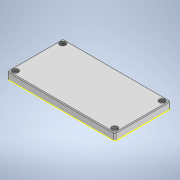
# Autodesk Inventor part: CustomLid_Rev3a
Saved by Autodesk Inventor 2021 (Build 250183000, 183)
## iProperties
Created: 2021-04-06
Part Number: CustomLid_Rev3a
Material: Generic
Document SubType Name: Modeling
Designer: James
Density: 1 g/cm^3
Appearance: Default
Author: James
Autodesk Inventor part; units mm, degrees
ref_plane "YZ Plane" through (0, 0, 0) normal (1, 0, 0) x (0, 1, 0)
ref_plane "XZ Plane" through (0, 0, 0) normal (0, 1, 0) x (-1, 0, 0)
ref_plane "XY Plane" through (0, 0, 0) normal (0, 0, 1) x (1, 0, 0)
sketch "Sketch1" plane through (0, 0, 0) normal (0, 1, 0) x (-1, 0, 0)
  line L0 (103.9624, -60.4464) -> (103.9624, 16.5536) projected
  arc A0 (103.9624, 16.5536) -> (101.9624, 18.5536) centre (101.9624, 16.5536) ccw projected
  line L1 (101.9624, 18.5536) -> (-50.0376, 18.5536) projected
  arc A1 (-50.0376, 18.5536) -> (-52.0376, 16.5536) centre (-50.0376, 16.5536) ccw projected
  line L2 (-52.0376, 16.5536) -> (-52.0376, -60.4464) projected
  arc A2 (-52.0376, -60.4464) -> (-50.0376, -62.4464) centre (-50.0376, -60.4464) ccw projected
  line L3 (-50.0376, -62.4464) -> (101.9624, -62.4464) projected
  arc A3 (101.9624, -62.4464) -> (103.9624, -60.4464) centre (101.9624, -60.4464) ccw projected
  arc A4 (97.8999, -50.5293) -> (92.0453, -56.3839) centre (97.7805, -56.2644) ccw projected
  arc A5 (97.8833, -51.3291) -> (92.8451, -56.3672) centre (97.7805, -56.2644) ccw projected
  circle A6 centre (97.7805, -56.2644) radius 2.5 projected
  arc A7 (97.8999, -50.5293) -> (100.9624, -47.5299) centre (97.9624, -47.5299) ccw projected
  arc A8 (97.8833, -51.3291) -> (101.7624, -47.5299) centre (97.9624, -47.5299) ccw projected
  line L4 (100.9624, 3.6371) -> (100.9624, -47.5299) projected
  line L5 (101.7624, -47.5299) -> (101.7624, 3.6371) projected
  arc A9 (89.046, -60.2464) -> (92.8451, -56.3672) centre (89.046, -56.4464) ccw projected
  arc A10 (89.046, -59.4464) -> (92.0453, -56.3839) centre (89.046, -56.4464) ccw projected
  line L6 (89.046, -59.4464) -> (-37.1211, -59.4464) projected
  line L7 (-37.1211, -60.2464) -> (89.046, -60.2464) projected
  circle A11 centre (-45.8556, -56.2644) radius 2.5 projected
  arc A12 (-40.9203, -56.3672) -> (-45.9584, -51.3291) centre (-45.8556, -56.2644) ccw projected
  arc A13 (-40.1204, -56.3839) -> (-45.9751, -50.5293) centre (-45.8556, -56.2644) ccw projected
  arc A14 (-40.1204, -56.3839) -> (-37.1211, -59.4464) centre (-37.1211, -56.4464) ccw projected
  arc A15 (-40.9203, -56.3672) -> (-37.1211, -60.2464) centre (-37.1211, -56.4464) ccw projected
  arc A16 (-49.0376, -47.5299) -> (-45.9751, -50.5293) centre (-46.0376, -47.5299) ccw projected
  arc A17 (-49.8376, -47.5299) -> (-45.9584, -51.3291) centre (-46.0376, -47.5299) ccw projected
  line L8 (-49.0376, -47.5299) -> (-49.0376, 3.6371) projected
  line L9 (-49.8376, 3.6371) -> (-49.8376, -47.5299) projected
  circle A18 centre (-45.8556, 12.3716) radius 2.5 projected
  arc A19 (-45.9584, 7.4363) -> (-40.9203, 12.4745) centre (-45.8556, 12.3716) ccw projected
  arc A20 (-45.9751, 6.6365) -> (-40.1204, 12.4911) centre (-45.8556, 12.3716) ccw projected
  arc A21 (-45.9584, 7.4363) -> (-49.8376, 3.6371) centre (-46.0376, 3.6371) ccw projected
  arc A22 (-45.9751, 6.6365) -> (-49.0376, 3.6371) centre (-46.0376, 3.6371) ccw projected
  line L10 (-49.0376, -47.5299) -> (-49.0376, 3.6371) projected
  line L11 (-49.8376, 3.6371) -> (-49.8376, -47.5299) projected
  arc A23 (-37.1211, 16.3536) -> (-40.9203, 12.4745) centre (-37.1211, 12.5536) ccw projected
  arc A24 (-37.1211, 15.5536) -> (-40.1204, 12.4911) centre (-37.1211, 12.5536) ccw projected
  line L12 (89.046, 16.3536) -> (-37.1211, 16.3536) projected
  line L13 (-37.1211, 15.5536) -> (89.046, 15.5536) projected
  circle A25 centre (97.7805, 12.3716) radius 2.5 projected
  arc A26 (100.9624, 3.6371) -> (97.8999, 6.6365) centre (97.9624, 3.6371) ccw projected
  arc A27 (101.7624, 3.6371) -> (97.8833, 7.4363) centre (97.9624, 3.6371) ccw projected
  arc A28 (92.8451, 12.4745) -> (97.8833, 7.4363) centre (97.7805, 12.3716) ccw projected
  arc A29 (92.0453, 12.4911) -> (97.8999, 6.6365) centre (97.7805, 12.3716) ccw projected
  arc A30 (92.0453, 12.4911) -> (89.046, 15.5536) centre (89.046, 12.5536) ccw projected
  arc A31 (92.8451, 12.4745) -> (89.046, 16.3536) centre (89.046, 12.5536) ccw projected
  arc A32 (-48.3376, -47.5299) -> (-45.9897, -49.8294) centre (-46.0376, -47.5299) ccw
  arc A33 (-39.4206, -56.3985) -> (-45.9897, -49.8294) centre (-45.8556, -56.2644) ccw
  arc A34 (-39.4206, -56.3985) -> (-37.1211, -58.7464) centre (-37.1211, -56.4464) ccw
  line L14 (-37.1211, -58.7464) -> (89.046, -58.7464)
  arc A35 (89.046, -58.7464) -> (91.3455, -56.3985) centre (89.046, -56.4464) ccw
  arc A36 (97.9145, -49.8294) -> (91.3455, -56.3985) centre (97.7805, -56.2644) ccw
  arc A37 (97.9145, -49.8294) -> (100.2624, -47.5299) centre (97.9624, -47.5299) ccw
  line L15 (100.2624, -47.5299) -> (100.2624, 3.6371)
  arc A38 (100.2624, 3.6371) -> (97.9145, 5.9366) centre (97.9624, 3.6371) ccw
  arc A39 (91.3455, 12.5057) -> (97.9145, 5.9366) centre (97.7805, 12.3716) ccw
  arc A40 (91.3455, 12.5057) -> (89.046, 14.8536) centre (89.046, 12.5536) ccw
  line L16 (89.046, 14.8536) -> (-37.1211, 14.8536)
  arc A41 (-37.1211, 14.8536) -> (-39.4206, 12.5057) centre (-37.1211, 12.5536) ccw
  arc A42 (-45.9897, 5.9366) -> (-39.4206, 12.5057) centre (-45.8556, 12.3716) ccw
  arc A43 (-45.9897, 5.9366) -> (-48.3376, 3.6371) centre (-46.0376, 3.6371) ccw
  arc A44 (-45.9438, 8.1362) -> (-50.5376, 3.6371) centre (-46.0376, 3.6371) ccw
  arc A45 (-45.9438, 8.1362) -> (-41.6201, 12.4599) centre (-45.8556, 12.3716) ccw
  arc A46 (-37.1211, 17.0536) -> (-41.6201, 12.4599) centre (-37.1211, 12.5536) ccw
  line L17 (-37.1211, 17.0536) -> (89.046, 17.0536)
  arc A47 (93.545, 12.4599) -> (89.046, 17.0536) centre (89.046, 12.5536) ccw
  arc A48 (93.545, 12.4599) -> (97.8687, 8.1362) centre (97.7805, 12.3716) ccw
  arc A49 (102.4624, 3.6371) -> (97.8687, 8.1362) centre (97.9624, 3.6371) ccw
  line L18 (102.4624, 3.6371) -> (102.4624, -47.5299)
  arc A50 (97.8687, -52.0289) -> (102.4624, -47.5299) centre (97.9624, -47.5299) ccw
  arc A51 (97.8687, -52.0289) -> (93.545, -56.3527) centre (97.7805, -56.2644) ccw
  arc A52 (89.046, -60.9464) -> (93.545, -56.3527) centre (89.046, -56.4464) ccw
  line L19 (89.046, -60.9464) -> (-37.1211, -60.9464)
  arc A53 (-41.6201, -56.3527) -> (-37.1211, -60.9464) centre (-37.1211, -56.4464) ccw
  arc A54 (-41.6201, -56.3527) -> (-45.9438, -52.0289) centre (-45.8556, -56.2644) ccw
  arc A55 (-50.5376, -47.5299) -> (-45.9438, -52.0289) centre (-46.0376, -47.5299) ccw
  line L20 (-48.3376, -47.5299) -> (-48.3376, 3.6371)
  line L21 (-50.5376, 3.6371) -> (-50.5376, -47.5299)
  line L22 (-37.1211, 13.8536) -> (89.046, 13.8536)
  arc A56 (90.3457, 12.5265) -> (89.046, 13.8536) centre (89.046, 12.5536) ccw
  arc A57 (90.3457, 12.5265) -> (97.9354, 4.9368) centre (97.7805, 12.3716) ccw
  arc A58 (99.2624, 3.6371) -> (97.9354, 4.9368) centre (97.9624, 3.6371) ccw
  line L23 (99.2624, 3.6371) -> (99.2624, -47.5299)
  arc A59 (97.9354, -48.8296) -> (99.2624, -47.5299) centre (97.9624, -47.5299) ccw
  arc A60 (97.9354, -48.8296) -> (90.3457, -56.4193) centre (97.7805, -56.2644) ccw
  arc A61 (89.046, -57.7464) -> (90.3457, -56.4193) centre (89.046, -56.4464) ccw
  line L24 (89.046, -57.7464) -> (-37.1211, -57.7464)
  arc A62 (-38.4208, -56.4193) -> (-37.1211, -57.7464) centre (-37.1211, -56.4464) ccw
  arc A63 (-38.4208, -56.4193) -> (-46.0105, -48.8296) centre (-45.8556, -56.2644) ccw
  arc A64 (-47.3376, -47.5299) -> (-46.0105, -48.8296) centre (-46.0376, -47.5299) ccw
  line L25 (-47.3376, -47.5299) -> (-47.3376, 3.6371)
  arc A65 (-46.0105, 4.9368) -> (-47.3376, 3.6371) centre (-46.0376, 3.6371) ccw
  arc A66 (-46.0105, 4.9368) -> (-38.4208, 12.5265) centre (-45.8556, 12.3716) ccw
  arc A67 (-37.1211, 13.8536) -> (-38.4208, 12.5265) centre (-37.1211, 12.5536) ccw
  circle A68 centre (-32.1211, -53.4464) radius 1.25
  circle A69 centre (-43.0376, -21.9464) radius 1.25
  circle A70 centre (-32.1211, 9.5536) radius 1.25
  circle A71 centre (25.9624, 9.5536) radius 1.25
  circle A72 centre (25.9624, -53.4464) radius 1.25
  circle A73 centre (84.046, -53.4464) radius 1.25
  circle A74 centre (94.9624, -21.9464) radius 1.25
  circle A75 centre (84.046, 9.5536) radius 1.25
  circle A76 centre (-32.1211, 9.5536) radius 2.25
  circle A77 centre (25.9624, 9.5536) radius 2.25
  circle A78 centre (25.9624, -53.4464) radius 2.25
  circle A79 centre (-32.1211, -53.4464) radius 2.25
  circle A80 centre (-43.0376, -21.9464) radius 2.25
  circle A81 centre (84.046, 9.5536) radius 2.25
  circle A82 centre (94.9624, -21.9464) radius 2.25
  circle A83 centre (84.046, -53.4464) radius 2.25
  point P0 (0, 0)
  dimension "lid_gasket_delta" = 0.7
  dimension "d1" = 0.7
  dimension "d2" = 0.7
  dimension "d3" = 0.7
  dimension "d8" = 1
  constraints: 72 point on circle, 52 centre point, 24 end point, 2 parallel, 75 other
  measures "lid_gasket_delta" distance between parallel lines of L6 L14
  measures "d1" distance between parallel lines of L7 L19
  measures "d2" distance between parallel lines of L8 L20
  measures "d3" distance between parallel lines of L9 L21
  measures "d8" distance between parallel lines of L16 L22
extrude "Extrusion1" add sketch "Sketch1" along normal blind 10 contours A3 L3 A2 L2 A1 L1 A0 L0 | A4 A10 L6 A14 A13 A16 L8 A22 A20 A24 L13 A30 A29 A26 L4 A7 | A5 A9 L7 A15 A12 A17 L9 A21 A19 A23 L12 A31 A28 A27 L5 A8 | A6 | A11 | A18 | A25 | L20 A43 A42 A41 L16 A40 A39 A38 L15 A37 A36 A35 L14 A34 A33 A32 | A45 A46 L17 A47 A48 A49 L18 A50 A51 A52 L19 A53 A54 A55 L21 A44 | L22 A56 A57 A58 L23 A59 A60 A61 L24 A62 A63 A64 L25 A65 A66 A67 | A68 | A69 | A70 | A71 | A72 | A73 | A74 | A75 | A76 | A77 | A78 | A79 | A80 | A81 | A82 | A83
extrude "Extrusion2" cut sketch "Sketch1" along normal blind 7 from surface at 0 contours L22 A56 A57 A58 L23 A59 A60 A61 L24 A62 A63 A64 L25 A65 A66 A67 | A68 | A69 | A70 | A71 | A72 | A73 | A74 | A75 | A76 | A77 | A78 | A79 | A80 | A81 | A82 | A83
extrude "Extrusion3" cut sketch "Sketch1" along normal blind 2.5 contours A4 A10 L6 A14 A13 A16 L8 A22 A20 A24 L13 A30 A29 A26 L4 A7 | A5 A9 L7 A15 A12 A17 L9 A21 A19 A23 L12 A31 A28 A27 L5 A8 | A45 A46 L17 A47 A48 A49 L18 A50 A51 A52 L19 A53 A54 A55 L21 A44
ref_plane "Bottom Face" through (5.5793, 7, -57.7464) normal (0, -1, 0) x (1, 0, 0)
sketch "Sketch2" plane through (5.5793, 7, -57.7464) normal (0, -1, 0) x (1, 0, 0)
  circle A0 centre (26.5418, 67.3) radius 2.25 projected
  circle A1 centre (26.5418, 67.3) radius 1.25 projected
  circle A2 centre (37.4582, 35.8) radius 2.25 projected
  circle A3 centre (37.4582, 35.8) radius 1.25 projected
  circle A4 centre (26.5418, 4.3) radius 2.25 projected
  circle A5 centre (26.5418, 4.3) radius 1.25 projected
  circle A6 centre (-31.5418, 67.3) radius 2.25 projected
  circle A7 centre (-31.5418, 67.3) radius 1.25 projected
  circle A8 centre (-31.5418, 4.3) radius 2.25 projected
  circle A9 centre (-31.5418, 4.3) radius 1.25 projected
  circle A10 centre (-89.6253, 67.3) radius 2.25 projected
  circle A11 centre (-89.6253, 67.3) radius 1.25 projected
  circle A12 centre (-89.6253, 4.3) radius 2.25 projected
  circle A13 centre (-89.6253, 4.3) radius 1.25 projected
  circle A14 centre (-100.5418, 35.8) radius 2.25 projected
  circle A15 centre (-100.5418, 35.8) radius 1.25 projected
extrude "Extrusion4" add sketch "Sketch2" along normal blind 4 contours A0 | A1 | A2 | A3 | A4 | A5 | A6 | A7 | A8 | A9 | A10 | A11 | A12 | A13 | A14 | A15
extrude "Extrusion5" cut sketch "Sketch2" along normal blind 4 contours A1 | A3 | A5 | A7 | A9 | A11 | A13 | A15
fillet "Fillet1" radius 1.5 8 edges at (-86.296, 7, 9.5536) (-28.2124, 7, 9.5536) (29.8711, 7, 9.5536) (40.7876, 7, -21.9464) (29.8711, 7, -53.4464) (-28.2124, 7, -53.4464) (-86.296, 7, -53.4464) (-97.2124, 7, -21.9464)
ref_plane "Top Face" through (50.0376, 10, -62.4464) normal (0, 1, 0) x (-1, 0, 0)
sketch "Sketch3" plane through (50.0376, 10, -62.4464) normal (0, 1, 0) x (-1, 0, 0)
  circle A0 centre (147.818, 74.818) radius 2.5 projected
  circle A1 centre (4.182, 74.818) radius 2.5 projected
  circle A2 centre (4.182, 6.182) radius 2.5 projected
  circle A3 centre (147.818, 6.182) radius 2.5 projected
  point P0 (50.0376, 62.4464)
  point P1 (148.052, 74.8409)
  point P2 (148.052, 6.3093)
hole "Hole1" at (45.8556, 10, 12.3716) at (45.8556, 10, -56.2644) at (-98.0144, 10, 12.3945) at (-98.0144, 10, -56.1371) direction (0, -1, 0) diameter 4 end through all counterbore diameter 7.5 counterbore depth 2.5
fillet "Fillet2" radius 0.5 4 edges at (45.8556, 10, 8.6216) (45.8556, 10, -60.0144) (-98.0144, 10, 8.6445) (-98.0144, 10, -59.8871)
fillet "Fillet3" radius 0.5 4 edges at (45.8556, 7.5, 8.6216) (45.8556, 7.5, -60.0144) (-98.0144, 7.5, 8.6445) (-98.0144, 7.5, -59.8871) inverted yes
ref_plane "Inspection Plane" through (45.8556, 0, 12.3716) normal (0, 0, 1) x (1, 0, 0)
sketch "Sketch4" plane through (45.8556, 0, 12.3716) normal (0, 0, 1) x (1, 0, 0)
  point P0 (-45.8556, 0)
ref_plane "Ceiling" through (5.5793, 7, -57.7464) normal (0, -1, 0) x (1, 0, 0)
sketch "Sketch5" plane through (5.5793, 7, -57.7464) normal (0, -1, 0) x (1, 0, 0)
  line L0 (-84.1448, 70.2927) -> (6.5043, 70.2927) construction
  line L1 (6.5043, 70.2927) -> (6.5043, 55.3746) construction
  line L2 (6.5043, 55.3746) -> (-84.1448, 55.3746) construction
  line L3 (-84.1448, 55.3746) -> (-84.1448, 70.2927) construction
  line L4 (-84.1654, 67.04) -> (-83.169, 68.6586)
  line L5 (-83.169, 68.6586) -> (-84.1654, 70.21)
  line L6 (-84.1654, 70.21) -> (-83.4116, 70.21)
  line L7 (-83.4116, 70.21) -> (-82.7637, 69.1026)
  line L8 (-82.7637, 69.1026) -> (-82.1209, 70.21)
  line L9 (-82.1209, 70.21) -> (-81.362, 70.21)
  line L10 (-81.362, 70.21) -> (-82.3584, 68.6638)
  line L11 (-82.3584, 68.6638) -> (-81.362, 67.04)
  line L12 (-81.362, 67.04) -> (-82.1158, 67.04)
  line L13 (-82.1158, 67.04) -> (-82.7637, 68.1372)
  line L14 (-82.7637, 68.1372) -> (-83.4116, 67.04)
  line L15 (-83.4116, 67.04) -> (-84.1654, 67.04)
  line L16 (-81.0574, 67.04) -> (-81.0574, 70.21)
  line L17 (-81.0574, 70.21) -> (-78.7547, 70.21)
  line L18 (-78.7547, 70.21) -> (-78.7547, 69.6576)
  line L19 (-78.7547, 69.6576) -> (-80.4146, 69.6576)
  line L20 (-80.4146, 69.6576) -> (-80.4146, 68.9813)
  line L21 (-80.4146, 68.9813) -> (-78.8967, 68.9813)
  line L22 (-78.8967, 68.9813) -> (-78.8967, 68.4392)
  line L23 (-78.8967, 68.4392) -> (-80.4146, 68.4392)
  line L24 (-80.4146, 68.4392) -> (-80.4146, 67.626)
  line L25 (-80.4146, 67.626) -> (-78.6773, 67.626)
  line L26 (-78.6773, 67.626) -> (-78.6773, 67.04)
  line L27 (-78.6773, 67.04) -> (-81.0574, 67.04)
  spline S0 degree 2 poles (-75.4195, 68.1294) (-75.4557, 67.5899) (-76.2172, 66.9523) (-76.8264, 66.9523) knots 0 0 0 1 2 2 2
  spline S1 degree 2 poles (-76.8264, 66.9523) (-77.5311, 66.9523) (-78.3133, 67.83) (-78.3133, 68.6225) knots 0 0 0 1 2 2 2
  spline S2 degree 2 poles (-78.3133, 68.6225) (-78.3133, 69.433) (-77.5157, 70.2927) (-76.7696, 70.2927) knots 0 0 0 1 2 2 2
  spline S3 degree 2 poles (-76.7696, 70.2927) (-76.163, 70.2927) (-75.4583, 69.6989) (-75.4247, 69.1594) knots 0 0 0 1 2 2 2
  line L28 (-75.4247, 69.1594) -> (-76.0675, 69.1594)
  spline S4 degree 2 poles (-76.0675, 69.1594) (-76.1088, 69.4305) (-76.465, 69.7118) (-76.7696, 69.7118) knots 0 0 0 1 2 2 2
  spline S5 degree 2 poles (-76.7696, 69.7118) (-77.2007, 69.7118) (-77.6473, 69.1568) (-77.6473, 68.6225) knots 0 0 0 1 2 2 2
  spline S6 degree 2 poles (-77.6473, 68.6225) (-77.6473, 68.1062) (-77.2007, 67.5434) (-76.7903, 67.5434) knots 0 0 0 1 2 2 2
  spline S7 degree 2 poles (-76.7903, 67.5434) (-76.4934, 67.5434) (-76.1165, 67.8455) (-76.0597, 68.1294) knots 0 0 0 1 2 2 2
  line L29 (-76.0597, 68.1294) -> (-75.4195, 68.1294)
  line L30 (-74.9187, 70.2204) -> (-74.2605, 70.2204)
  line L31 (-74.2605, 70.2204) -> (-74.2605, 68.2327)
  spline S8 degree 2 poles (-74.2605, 68.2327) (-74.2605, 67.8635) (-73.9688, 67.5254) (-73.6487, 67.5254) knots 0 0 0 1 2 2 2
  spline S9 degree 2 poles (-73.6487, 67.5254) (-73.326, 67.5254) (-73.0317, 67.8609) (-73.0317, 68.2327) knots 0 0 0 1 2 2 2
  line L32 (-73.0317, 68.2327) -> (-73.0317, 70.2204)
  line L33 (-73.0317, 70.2204) -> (-72.3786, 70.2204)
  line L34 (-72.3786, 70.2204) -> (-72.3786, 68.1604)
  spline S10 degree 2 poles (-72.3786, 68.1604) (-72.3786, 67.577) (-73.0317, 66.9523) (-73.6435, 66.9523) knots 0 0 0 1 2 2 2
  spline S11 degree 2 poles (-73.6435, 66.9523) (-74.263, 66.9523) (-74.9187, 67.5744) (-74.9187, 68.1604) knots 0 0 0 1 2 2 2
  line L35 (-74.9187, 68.1604) -> (-74.9187, 70.2204)
  line L36 (-71.0801, 67.04) -> (-71.0801, 69.6447)
  line L37 (-71.0801, 69.6447) -> (-72.0198, 69.6447)
  line L38 (-72.0198, 69.6447) -> (-72.0198, 70.21)
  line L39 (-72.0198, 70.21) -> (-69.4926, 70.21)
  line L40 (-69.4926, 70.21) -> (-69.4926, 69.6447)
  line L41 (-69.4926, 69.6447) -> (-70.427, 69.6447)
  line L42 (-70.427, 69.6447) -> (-70.427, 67.04)
  line L43 (-70.427, 67.04) -> (-71.0801, 67.04)
  line L44 (-69.1157, 67.04) -> (-69.1157, 70.21)
  line L45 (-69.1157, 70.21) -> (-66.813, 70.21)
  line L46 (-66.813, 70.21) -> (-66.813, 69.6576)
  line L47 (-66.813, 69.6576) -> (-68.4729, 69.6576)
  line L48 (-68.4729, 69.6576) -> (-68.4729, 68.9813)
  line L49 (-68.4729, 68.9813) -> (-66.955, 68.9813)
  line L50 (-66.955, 68.9813) -> (-66.955, 68.4392)
  line L51 (-66.955, 68.4392) -> (-68.4729, 68.4392)
  line L52 (-68.4729, 68.4392) -> (-68.4729, 67.626)
  line L53 (-68.4729, 67.626) -> (-66.7356, 67.626)
  line L54 (-66.7356, 67.626) -> (-66.7356, 67.04)
  line L55 (-66.7356, 67.04) -> (-69.1157, 67.04)
  line L56 (-64.2368, 67.04) -> (-65.3313, 70.21)
  line L57 (-65.3313, 70.21) -> (-64.6085, 70.21)
  line L58 (-64.6085, 70.21) -> (-63.9322, 67.8377)
  line L59 (-63.9322, 67.8377) -> (-63.2455, 70.21)
  line L60 (-63.2455, 70.21) -> (-62.5304, 70.21)
  line L61 (-62.5304, 70.21) -> (-63.6121, 67.04)
  line L62 (-63.6121, 67.04) -> (-64.2368, 67.04)
  line L63 (-60.8396, 67.7499) -> (-60.2149, 67.7499)
  spline S12 degree 2 poles (-60.2149, 67.7499) (-60.3104, 67.3808) (-60.8835, 66.96) (-61.2965, 66.96) knots 0 0 0 1 2 2 2
  spline S13 degree 2 poles (-61.2965, 66.96) (-61.8051, 66.96) (-62.3988, 67.6415) (-62.3988, 68.2249) knots 0 0 0 1 2 2 2
  spline S14 degree 2 poles (-62.3988, 68.2249) (-62.3988, 68.8006) (-61.8128, 69.464) (-61.3043, 69.464) knots 0 0 0 1 2 2 2
  spline S15 degree 2 poles (-61.3043, 69.464) (-60.7673, 69.464) (-60.1813, 68.8109) (-60.1813, 68.2069) knots 0 0 0 1 2 2 2
  spline S16 degree 2 poles (-60.1813, 68.2069) (-60.1813, 68.1423) (-60.1839, 68.0752) (-60.1891, 68.0442) knots 0 0 0 1 2 2 2
  line L64 (-60.1891, 68.0442) -> (-61.7508, 68.0442)
  spline S17 degree 2 poles (-61.7508, 68.0442) (-61.7379, 67.768) (-61.4953, 67.4892) (-61.2681, 67.4892) knots 0 0 0 1 2 2 2
  spline S18 degree 2 poles (-61.2681, 67.4892) (-61.1055, 67.4892) (-60.899, 67.6157) (-60.8396, 67.7499) knots 0 0 0 1 2 2 2
  line L65 (-61.7508, 68.4547) -> (-60.8293, 68.4547)
  spline S19 degree 2 poles (-60.8293, 68.4547) (-60.837, 68.6922) (-61.0719, 68.94) (-61.2913, 68.94) knots 0 0 0 1 2 2 2
  spline S20 degree 2 poles (-61.2913, 68.94) (-61.4979, 68.94) (-61.7302, 68.6896) (-61.7508, 68.4547) knots 0 0 0 1 2 2 2
  line L66 (-59.7657, 67.04) -> (-59.7657, 69.3814)
  line L67 (-59.7657, 69.3814) -> (-59.1513, 69.3814)
  line L68 (-59.1513, 69.3814) -> (-59.1513, 69.1026)
  spline S21 degree 2 poles (-59.1513, 69.1026) (-59.0197, 69.273) (-58.6634, 69.4434) (-58.444, 69.4434) knots 0 0 0 1 2 2 2
  spline S22 degree 2 poles (-58.444, 69.4434) (-58.0568, 69.4434) (-57.6722, 69.0407) (-57.6722, 68.6354) knots 0 0 0 1 2 2 2
  line L69 (-57.6722, 68.6354) -> (-57.6722, 67.04)
  line L70 (-57.6722, 67.04) -> (-58.2995, 67.04)
  line L71 (-58.2995, 67.04) -> (-58.2995, 68.4547)
  spline S23 degree 2 poles (-58.2995, 68.4547) (-58.2995, 68.7077) (-58.4698, 68.9219) (-58.6609, 68.9219) knots 0 0 0 1 2 2 2
  spline S24 degree 2 poles (-58.6609, 68.9219) (-58.8803, 68.9219) (-59.1384, 68.656) (-59.1384, 68.4289) knots 0 0 0 1 2 2 2
  line L72 (-59.1384, 68.4289) -> (-59.1384, 67.04)
  line L73 (-59.1384, 67.04) -> (-59.7657, 67.04)
  spline S25 degree 2 poles (-56.0949, 67.022) (-56.1801, 67.0194) (-56.4202, 67.0091) (-56.4512, 67.0091) knots 0 0 0 1 2 2 2
  spline S26 degree 2 poles (-56.4512, 67.0091) (-56.81, 67.0091) (-57.0759, 67.2775) (-57.0759, 67.6751) knots 0 0 0 1 2 2 2
  line L74 (-57.0759, 67.6751) -> (-57.0759, 68.9426)
  line L75 (-57.0759, 68.9426) -> (-57.3856, 68.9426)
  line L76 (-57.3856, 68.9426) -> (-57.3856, 69.3814)
  line L77 (-57.3856, 69.3814) -> (-57.0759, 69.3814)
  line L78 (-57.0759, 69.3814) -> (-57.0759, 70.019)
  line L79 (-57.0759, 70.019) -> (-56.4563, 70.019)
  line L80 (-56.4563, 70.019) -> (-56.4563, 69.3814)
  line L81 (-56.4563, 69.3814) -> (-56.0949, 69.3814)
  line L82 (-56.0949, 69.3814) -> (-56.0949, 68.9426)
  line L83 (-56.0949, 68.9426) -> (-56.4563, 68.9426)
  line L84 (-56.4563, 68.9426) -> (-56.4563, 67.6441)
  spline S27 degree 2 poles (-56.4563, 67.6441) (-56.4563, 67.5538) (-56.3737, 67.4944) (-56.2472, 67.4944) knots 0 0 0 1 2 2 2
  line L85 (-56.2472, 67.4944) -> (-56.0949, 67.4944)
  line L86 (-56.0949, 67.4944) -> (-56.0949, 67.022)
  line L87 (-53.6451, 69.3814) -> (-53.6451, 67.04)
  line L88 (-53.6451, 67.04) -> (-54.2595, 67.04)
  line L89 (-54.2595, 67.04) -> (-54.2595, 67.3188)
  spline S28 degree 2 poles (-54.2595, 67.3188) (-54.3938, 67.1485) (-54.7474, 66.9781) (-54.9694, 66.9781) knots 0 0 0 1 2 2 2
  spline S29 degree 2 poles (-54.9694, 66.9781) (-55.3541, 66.9781) (-55.7387, 67.3834) (-55.7387, 67.7861) knots 0 0 0 1 2 2 2
  line L90 (-55.7387, 67.7861) -> (-55.7387, 69.3814)
  line L91 (-55.7387, 69.3814) -> (-55.1114, 69.3814)
  line L92 (-55.1114, 69.3814) -> (-55.1114, 67.9668)
  spline S30 degree 2 poles (-55.1114, 67.9668) (-55.1114, 67.719) (-54.9436, 67.5047) (-54.75, 67.5047) knots 0 0 0 1 2 2 2
  spline S31 degree 2 poles (-54.75, 67.5047) (-54.5332, 67.5047) (-54.2724, 67.7706) (-54.2724, 67.9978) knots 0 0 0 1 2 2 2
  line L93 (-54.2724, 67.9978) -> (-54.2724, 69.3814)
  line L94 (-54.2724, 69.3814) -> (-53.6451, 69.3814)
  line L95 (-53.0979, 67.04) -> (-53.0979, 69.3814)
  line L96 (-53.0979, 69.3814) -> (-52.5171, 69.3814)
  line L97 (-52.5171, 69.3814) -> (-52.5171, 68.9787)
  spline S32 degree 2 poles (-52.5171, 68.9787) (-52.3931, 69.2188) (-52.0653, 69.4459) (-51.8407, 69.4459) knots 0 0 0 1 2 2 2
  spline S33 degree 2 poles (-51.8407, 69.4459) (-51.8046, 69.4459) (-51.7633, 69.4434) (-51.7504, 69.4408) knots 0 0 0 1 2 2 2
  line L98 (-51.7504, 69.4408) -> (-51.7478, 68.8057)
  line L99 (-51.7478, 68.8057) -> (-51.9569, 68.8057)
  spline S34 degree 2 poles (-51.9569, 68.8057) (-52.2124, 68.8057) (-52.4706, 68.5399) (-52.4706, 68.2766) knots 0 0 0 1 2 2 2
  line L100 (-52.4706, 68.2766) -> (-52.4706, 67.04)
  line L101 (-52.4706, 67.04) -> (-53.0979, 67.04)
  line L102 (-49.964, 67.7499) -> (-49.3393, 67.7499)
  spline S35 degree 2 poles (-49.3393, 67.7499) (-49.4348, 67.3808) (-50.0079, 66.96) (-50.4209, 66.96) knots 0 0 0 1 2 2 2
  spline S36 degree 2 poles (-50.4209, 66.96) (-50.9295, 66.96) (-51.5232, 67.6415) (-51.5232, 68.2249) knots 0 0 0 1 2 2 2
  spline S37 degree 2 poles (-51.5232, 68.2249) (-51.5232, 68.8006) (-50.9372, 69.464) (-50.4287, 69.464) knots 0 0 0 1 2 2 2
  spline S38 degree 2 poles (-50.4287, 69.464) (-49.8917, 69.464) (-49.3058, 68.8109) (-49.3058, 68.2069) knots 0 0 0 1 2 2 2
  spline S39 degree 2 poles (-49.3058, 68.2069) (-49.3058, 68.1423) (-49.3083, 68.0752) (-49.3135, 68.0442) knots 0 0 0 1 2 2 2
  line L103 (-49.3135, 68.0442) -> (-50.8753, 68.0442)
  spline S40 degree 2 poles (-50.8753, 68.0442) (-50.8624, 67.768) (-50.6197, 67.4892) (-50.3925, 67.4892) knots 0 0 0 1 2 2 2
  spline S41 degree 2 poles (-50.3925, 67.4892) (-50.2299, 67.4892) (-50.0234, 67.6157) (-49.964, 67.7499) knots 0 0 0 1 2 2 2
  line L104 (-50.8753, 68.4547) -> (-49.9537, 68.4547)
  spline S42 degree 2 poles (-49.9537, 68.4547) (-49.9614, 68.6922) (-50.1963, 68.94) (-50.4158, 68.94) knots 0 0 0 1 2 2 2
  spline S43 degree 2 poles (-50.4158, 68.94) (-50.6223, 68.94) (-50.8546, 68.6896) (-50.8753, 68.4547) knots 0 0 0 1 2 2 2
  line L105 (-49.0218, 67.8016) -> (-48.3971, 67.8016)
  spline S44 degree 2 poles (-48.3971, 67.8016) (-48.3893, 67.6235) (-48.1467, 67.4479) (-47.9066, 67.4479) knots 0 0 0 1 2 2 2
  spline S45 degree 2 poles (-47.9066, 67.4479) (-47.7233, 67.4479) (-47.522, 67.5718) (-47.522, 67.6828) knots 0 0 0 1 2 2 2
  spline S46 degree 2 poles (-47.522, 67.6828) (-47.522, 67.8429) (-47.8963, 67.9229) knots 0 0 0 1 1 1
  spline S47 degree 2 poles (-47.8963, 67.9229) (-48.0486, 67.9539) (-48.1389, 67.9771) knots 0 0 0 1 1 1
  spline S48 degree 2 poles (-48.1389, 67.9771) (-48.5959, 68.0933) (-48.9521, 68.4134) (-48.9521, 68.6844) knots 0 0 0 1 2 2 2
  spline S49 degree 2 poles (-48.9521, 68.6844) (-48.9521, 69.0432) (-48.4332, 69.464) (-47.9892, 69.464) knots 0 0 0 1 2 2 2
  spline S50 degree 2 poles (-47.9892, 69.464) (-47.5194, 69.464) (-46.985, 69.0458) (-46.967, 68.6663) knots 0 0 0 1 2 2 2
  line L106 (-46.967, 68.6663) -> (-47.5762, 68.6663)
  spline S51 degree 2 poles (-47.5762, 68.6663) (-47.5814, 68.8161) (-47.7956, 68.9787) (-47.9841, 68.9787) knots 0 0 0 1 2 2 2
  spline S52 degree 2 poles (-47.9841, 68.9787) (-48.1622, 68.9787) (-48.3377, 68.8703) (-48.3377, 68.7644) knots 0 0 0 1 2 2 2
  spline S53 degree 2 poles (-48.3377, 68.7644) (-48.3377, 68.6225) (-47.8705, 68.5166) knots 0 0 0 1 1 1
  spline S54 degree 2 poles (-47.8705, 68.5166) (-47.7621, 68.4934) (-47.7001, 68.4779) knots 0 0 0 1 1 1
  spline S55 degree 2 poles (-47.7001, 68.4779) (-47.2329, 68.3669) (-46.8921, 68.0571) (-46.8921, 67.7758) knots 0 0 0 1 2 2 2
  spline S56 degree 2 poles (-46.8921, 67.7758) (-46.8921, 67.3782) (-47.4549, 66.96) (-47.9892, 66.96) knots 0 0 0 1 2 2 2
  spline S57 degree 2 poles (-47.9892, 66.96) (-48.4745, 66.96) (-49.0218, 67.3937) (-49.0218, 67.7758) knots 0 0 0 1 2 2 2
  line L107 (-49.0218, 67.7758) -> (-49.0218, 67.8016)
  line L108 (-45.1729, 67.04) -> (-45.1729, 70.21)
  line L109 (-45.1729, 70.21) -> (-44.5198, 70.21)
  line L110 (-44.5198, 70.21) -> (-44.5198, 67.626)
  line L111 (-44.5198, 67.626) -> (-42.9735, 67.626)
  line L112 (-42.9735, 67.626) -> (-42.9735, 67.04)
  line L113 (-42.9735, 67.04) -> (-45.1729, 67.04)
  line L114 (-42.6147, 67.04) -> (-42.6147, 70.21)
  line L115 (-42.6147, 70.21) -> (-41.9616, 70.21)
  line L116 (-41.9616, 70.21) -> (-41.9616, 67.626)
  line L117 (-41.9616, 67.626) -> (-40.4153, 67.626)
  line L118 (-40.4153, 67.626) -> (-40.4153, 67.04)
  line L119 (-40.4153, 67.04) -> (-42.6147, 67.04)
  spline S58 degree 2 poles (-37.2969, 68.1294) (-37.3331, 67.5899) (-38.0946, 66.9523) (-38.7038, 66.9523) knots 0 0 0 1 2 2 2
  spline S59 degree 2 poles (-38.7038, 66.9523) (-39.4085, 66.9523) (-40.1907, 67.83) (-40.1907, 68.6225) knots 0 0 0 1 2 2 2
  spline S60 degree 2 poles (-40.1907, 68.6225) (-40.1907, 69.433) (-39.393, 70.2927) (-38.647, 70.2927) knots 0 0 0 1 2 2 2
  spline S61 degree 2 poles (-38.647, 70.2927) (-38.0404, 70.2927) (-37.3356, 69.6989) (-37.3021, 69.1594) knots 0 0 0 1 2 2 2
  line L120 (-37.3021, 69.1594) -> (-37.9449, 69.1594)
  spline S62 degree 2 poles (-37.9449, 69.1594) (-37.9862, 69.4305) (-38.3424, 69.7118) (-38.647, 69.7118) knots 0 0 0 1 2 2 2
  spline S63 degree 2 poles (-38.647, 69.7118) (-39.0781, 69.7118) (-39.5247, 69.1568) (-39.5247, 68.6225) knots 0 0 0 1 2 2 2
  spline S64 degree 2 poles (-39.5247, 68.6225) (-39.5247, 68.1062) (-39.0781, 67.5434) (-38.6677, 67.5434) knots 0 0 0 1 2 2 2
  spline S65 degree 2 poles (-38.6677, 67.5434) (-38.3708, 67.5434) (-37.9939, 67.8455) (-37.9371, 68.1294) knots 0 0 0 1 2 2 2
  line L121 (-37.9371, 68.1294) -> (-37.2969, 68.1294)
  line L122 (-83.8582, 60.726) -> (-83.8582, 64.007)
  line L123 (-83.8582, 64.007) -> (-83.2619, 64.007)
  line L124 (-83.2619, 64.007) -> (-83.2619, 63.6869)
  spline S66 degree 2 poles (-83.2619, 63.6869) (-83.1251, 63.896) (-82.7921, 64.0844) (-82.5649, 64.0844) knots 0 0 0 1 2 2 2
  spline S67 degree 2 poles (-82.5649, 64.0844) (-82.1338, 64.0844) (-81.5943, 63.4029) (-81.5943, 62.8479) knots 0 0 0 1 2 2 2
  spline S68 degree 2 poles (-81.5943, 62.8479) (-81.5943, 62.2852) (-82.1338, 61.5856) (-82.5572, 61.5856) knots 0 0 0 1 2 2 2
  spline S69 degree 2 poles (-82.5572, 61.5856) (-82.7818, 61.5856) (-83.1329, 61.774) (-83.249, 61.9547) knots 0 0 0 1 2 2 2
  line L125 (-83.249, 61.9547) -> (-83.249, 60.726)
  line L126 (-83.249, 60.726) -> (-83.8582, 60.726)
  spline S70 degree 2 poles (-82.2164, 62.8195) (-82.2164, 63.1732) (-82.4849, 63.5449) (-82.7379, 63.5449) knots 0 0 0 1 2 2 2
  spline S71 degree 2 poles (-82.7379, 63.5449) (-82.9883, 63.5449) (-83.249, 63.1758) (-83.249, 62.8195) knots 0 0 0 1 2 2 2
  spline S72 degree 2 poles (-83.249, 62.8195) (-83.249, 62.4891) (-82.9754, 62.1277) (-82.725, 62.1277) knots 0 0 0 1 2 2 2
  spline S73 degree 2 poles (-82.725, 62.1277) (-82.4875, 62.1277) (-82.2164, 62.4968) (-82.2164, 62.8195) knots 0 0 0 1 2 2 2
  line L127 (-81.4239, 61.2552) -> (-80.3552, 64.9182)
  line L128 (-80.3552, 64.9182) -> (-80.0609, 64.9182)
  line L129 (-80.0609, 64.9182) -> (-81.1322, 61.2552)
  line L130 (-81.1322, 61.2552) -> (-81.4239, 61.2552)
  line L131 (-79.7718, 61.6656) -> (-79.7718, 64.007)
  line L132 (-79.7718, 64.007) -> (-79.1574, 64.007)
  line L133 (-79.1574, 64.007) -> (-79.1574, 63.7282)
  spline S74 degree 2 poles (-79.1574, 63.7282) (-79.0258, 63.8986) (-78.6696, 64.0689) (-78.4501, 64.0689) knots 0 0 0 1 2 2 2
  spline S75 degree 2 poles (-78.4501, 64.0689) (-78.0629, 64.0689) (-77.6783, 63.6662) (-77.6783, 63.2609) knots 0 0 0 1 2 2 2
  line L134 (-77.6783, 63.2609) -> (-77.6783, 61.6656)
  line L135 (-77.6783, 61.6656) -> (-78.3056, 61.6656)
  line L136 (-78.3056, 61.6656) -> (-78.3056, 63.0802)
  spline S76 degree 2 poles (-78.3056, 63.0802) (-78.3056, 63.3332) (-78.4759, 63.5475) (-78.667, 63.5475) knots 0 0 0 1 2 2 2
  spline S77 degree 2 poles (-78.667, 63.5475) (-78.8864, 63.5475) (-79.1445, 63.2816) (-79.1445, 63.0544) knots 0 0 0 1 2 2 2
  line L137 (-79.1445, 63.0544) -> (-79.1445, 61.6656)
  line L138 (-79.1445, 61.6656) -> (-79.7718, 61.6656)
  line L139 (-76.1785, 61.6656) -> (-75.182, 63.2842)
  line L140 (-75.182, 63.2842) -> (-76.1785, 64.8356)
  line L141 (-76.1785, 64.8356) -> (-75.4247, 64.8356)
  line L142 (-75.4247, 64.8356) -> (-74.7768, 63.7282)
  line L143 (-74.7768, 63.7282) -> (-74.134, 64.8356)
  line L144 (-74.134, 64.8356) -> (-73.375, 64.8356)
  line L145 (-73.375, 64.8356) -> (-74.3715, 63.2893)
  line L146 (-74.3715, 63.2893) -> (-73.375, 61.6656)
  line L147 (-73.375, 61.6656) -> (-74.1288, 61.6656)
  line L148 (-74.1288, 61.6656) -> (-74.7768, 62.7627)
  line L149 (-74.7768, 62.7627) -> (-75.4247, 61.6656)
  line L150 (-75.4247, 61.6656) -> (-76.1785, 61.6656)
  spline S78 degree 2 poles (-70.3109, 62.755) (-70.347, 62.2155) (-71.1085, 61.5779) (-71.7178, 61.5779) knots 0 0 0 1 2 2 2
  spline S79 degree 2 poles (-71.7178, 61.5779) (-72.4225, 61.5779) (-73.2047, 62.4555) (-73.2047, 63.248) knots 0 0 0 1 2 2 2
  spline S80 degree 2 poles (-73.2047, 63.248) (-73.2047, 64.0586) (-72.407, 64.9182) (-71.661, 64.9182) knots 0 0 0 1 2 2 2
  spline S81 degree 2 poles (-71.661, 64.9182) (-71.0543, 64.9182) (-70.3496, 64.3245) (-70.316, 63.785) knots 0 0 0 1 2 2 2
  line L151 (-70.316, 63.785) -> (-70.9588, 63.785)
  spline S82 degree 2 poles (-70.9588, 63.785) (-71.0001, 64.056) (-71.3564, 64.3374) (-71.661, 64.3374) knots 0 0 0 1 2 2 2
  spline S83 degree 2 poles (-71.661, 64.3374) (-72.0921, 64.3374) (-72.5387, 63.7824) (-72.5387, 63.248) knots 0 0 0 1 2 2 2
  spline S84 degree 2 poles (-72.5387, 63.248) (-72.5387, 62.7318) (-72.0921, 62.169) (-71.6816, 62.169) knots 0 0 0 1 2 2 2
  spline S85 degree 2 poles (-71.6816, 62.169) (-71.3848, 62.169) (-71.0079, 62.471) (-70.9511, 62.755) knots 0 0 0 1 2 2 2
  line L152 (-70.9511, 62.755) -> (-70.3109, 62.755)
  line L153 (-69.9856, 62.5433) -> (-69.9856, 63.1345)
  line L154 (-69.9856, 63.1345) -> (-68.7749, 63.1345)
  line L155 (-68.7749, 63.1345) -> (-68.7749, 62.5433)
  line L156 (-68.7749, 62.5433) -> (-69.9856, 62.5433)
  spline S86 degree 2 poles (-68.54, 61.6656) (-68.5348, 62.0787) (-68.1915, 62.6543) (-67.7527, 62.9486) knots 0 0 0 1 2 2 2
  spline S87 degree 2 poles (-67.7527, 62.9486) (-67.6856, 62.9951) (-67.5591, 63.0725) knots 0 0 0 1 1 1
  spline S88 degree 2 poles (-67.5591, 63.0725) (-66.9782, 63.4468) (-66.9782, 63.7901) knots 0 0 0 1 1 1
  spline S89 degree 2 poles (-66.9782, 63.7901) (-66.9782, 63.9941) (-67.2235, 64.2316) (-67.4352, 64.2316) knots 0 0 0 1 2 2 2
  spline S90 degree 2 poles (-67.4352, 64.2316) (-67.6675, 64.2316) (-67.9205, 63.9399) (-67.9205, 63.6714) knots 0 0 0 1 2 2 2
  line L157 (-67.9205, 63.6714) -> (-67.9205, 63.6456)
  line L158 (-67.9205, 63.6456) -> (-68.4884, 63.6456)
  spline S91 degree 2 poles (-68.4884, 63.6456) (-68.4884, 64.1748) (-67.9205, 64.7479) (-67.3939, 64.7479) knots 0 0 0 1 2 2 2
  spline S92 degree 2 poles (-67.3939, 64.7479) (-66.9189, 64.7479) (-66.351, 64.229) (-66.351, 63.8005) knots 0 0 0 1 2 2 2
  spline S93 degree 2 poles (-66.351, 63.8005) (-66.351, 63.4907) (-66.6478, 63.0389) (-67.0738, 62.7524) knots 0 0 0 1 2 2 2
  spline S94 degree 2 poles (-67.0738, 62.7524) (-67.1641, 62.6905) (-67.3242, 62.5872) knots 0 0 0 1 1 1
  spline S95 degree 2 poles (-67.3242, 62.5872) (-67.7294, 62.3291) (-67.7811, 62.1922) knots 0 0 0 1 1 1
  line L159 (-67.7811, 62.1922) -> (-66.3819, 62.1922)
  line L160 (-66.3819, 62.1922) -> (-66.3819, 61.6656)
  line L161 (-66.3819, 61.6656) -> (-68.54, 61.6656)
  line L162 (-64.7427, 61.6656) -> (-64.7427, 62.3316)
  line L163 (-64.7427, 62.3316) -> (-66.0412, 62.3316)
  line L164 (-66.0412, 62.3316) -> (-66.0412, 62.8737)
  line L165 (-66.0412, 62.8737) -> (-64.9054, 64.6601)
  line L166 (-64.9054, 64.6601) -> (-64.1412, 64.6601)
  line L167 (-64.1412, 64.6601) -> (-64.1412, 62.8221)
  line L168 (-64.1412, 62.8221) -> (-63.7824, 62.8221)
  line L169 (-63.7824, 62.8221) -> (-63.7824, 62.3316)
  line L170 (-63.7824, 62.3316) -> (-64.1412, 62.3316)
  line L171 (-64.1412, 62.3316) -> (-64.1412, 61.6656)
  line L172 (-64.1412, 61.6656) -> (-64.7427, 61.6656)
  line L173 (-64.7298, 62.8066) -> (-64.7298, 64.1257)
  line L174 (-64.7298, 64.1257) -> (-65.5662, 62.8066)
  line L175 (-65.5662, 62.8066) -> (-64.7298, 62.8066)
  line L176 (-62.5562, 61.6656) -> (-62.5562, 63.7721)
  line L177 (-62.5562, 63.7721) -> (-63.292, 63.7721)
  line L178 (-63.292, 63.7721) -> (-63.292, 64.2058)
  line L179 (-63.292, 64.2058) -> (-63.2455, 64.2058)
  spline S96 degree 2 poles (-63.2455, 64.2058) (-62.8428, 64.2058) (-62.4736, 64.4562) (-62.4427, 64.7479) knots 0 0 0 1 2 2 2
  line L180 (-62.4427, 64.7479) -> (-61.9496, 64.7479)
  line L181 (-61.9496, 64.7479) -> (-61.9496, 61.6656)
  line L182 (-61.9496, 61.6656) -> (-62.5562, 61.6656)
  line L183 (-61.0074, 62.5433) -> (-61.0074, 63.1345)
  line L184 (-61.0074, 63.1345) -> (-59.7967, 63.1345)
  line L185 (-59.7967, 63.1345) -> (-59.7967, 62.5433)
  line L186 (-59.7967, 62.5433) -> (-61.0074, 62.5433)
  spline S97 degree 2 poles (-59.5282, 63.1629) (-59.5282, 63.9579) (-58.9758, 64.7479) (-58.4156, 64.7479) knots 0 0 0 1 2 2 2
  spline S98 degree 2 poles (-58.4156, 64.7479) (-57.858, 64.7479) (-57.3005, 63.9528) (-57.3005, 63.1577) knots 0 0 0 1 2 2 2
  spline S99 degree 2 poles (-57.3005, 63.1577) (-57.3005, 62.3652) (-57.8529, 61.5804) (-58.4156, 61.5804) knots 0 0 0 1 2 2 2
  spline S100 degree 2 poles (-58.4156, 61.5804) (-58.9758, 61.5804) (-59.5282, 62.3678) (-59.5282, 63.1629) knots 0 0 0 1 2 2 2
  spline S101 degree 2 poles (-58.888, 63.1629) (-58.888, 62.6027) (-58.6634, 62.0941) (-58.4156, 62.0941) knots 0 0 0 1 2 2 2
  spline S102 degree 2 poles (-58.4156, 62.0941) (-58.1678, 62.0941) (-57.9406, 62.6053) (-57.9406, 63.1629) knots 0 0 0 1 2 2 2
  spline S103 degree 2 poles (-57.9406, 63.1629) (-57.9406, 63.723) (-58.1678, 64.2316) (-58.4156, 64.2316) knots 0 0 0 1 2 2 2
  spline S104 degree 2 poles (-58.4156, 64.2316) (-58.6634, 64.2316) (-58.888, 63.7256) (-58.888, 63.1629) knots 0 0 0 1 2 2 2
  spline S105 degree 2 poles (-57.0268, 63.1629) (-57.0268, 63.9579) (-56.4744, 64.7479) (-55.9142, 64.7479) knots 0 0 0 1 2 2 2
  spline S106 degree 2 poles (-55.9142, 64.7479) (-55.3566, 64.7479) (-54.799, 63.9528) (-54.799, 63.1577) knots 0 0 0 1 2 2 2
  spline S107 degree 2 poles (-54.799, 63.1577) (-54.799, 62.3652) (-55.3515, 61.5804) (-55.9142, 61.5804) knots 0 0 0 1 2 2 2
  spline S108 degree 2 poles (-55.9142, 61.5804) (-56.4744, 61.5804) (-57.0268, 62.3678) (-57.0268, 63.1629) knots 0 0 0 1 2 2 2
  spline S109 degree 2 poles (-56.3866, 63.1629) (-56.3866, 62.6027) (-56.162, 62.0941) (-55.9142, 62.0941) knots 0 0 0 1 2 2 2
  spline S110 degree 2 poles (-55.9142, 62.0941) (-55.6664, 62.0941) (-55.4392, 62.6053) (-55.4392, 63.1629) knots 0 0 0 1 2 2 2
  spline S111 degree 2 poles (-55.4392, 63.1629) (-55.4392, 63.723) (-55.6664, 64.2316) (-55.9142, 64.2316) knots 0 0 0 1 2 2 2
  spline S112 degree 2 poles (-55.9142, 64.2316) (-56.162, 64.2316) (-56.3866, 63.7256) (-56.3866, 63.1629) knots 0 0 0 1 2 2 2
  spline S113 degree 2 poles (-54.5254, 63.1629) (-54.5254, 63.9579) (-53.973, 64.7479) (-53.4128, 64.7479) knots 0 0 0 1 2 2 2
  spline S114 degree 2 poles (-53.4128, 64.7479) (-52.8552, 64.7479) (-52.2976, 63.9528) (-52.2976, 63.1577) knots 0 0 0 1 2 2 2
  spline S115 degree 2 poles (-52.2976, 63.1577) (-52.2976, 62.3652) (-52.8501, 61.5804) (-53.4128, 61.5804) knots 0 0 0 1 2 2 2
  spline S116 degree 2 poles (-53.4128, 61.5804) (-53.973, 61.5804) (-54.5254, 62.3678) (-54.5254, 63.1629) knots 0 0 0 1 2 2 2
  spline S117 degree 2 poles (-53.8852, 63.1629) (-53.8852, 62.6027) (-53.6606, 62.0941) (-53.4128, 62.0941) knots 0 0 0 1 2 2 2
  spline S118 degree 2 poles (-53.4128, 62.0941) (-53.165, 62.0941) (-52.9378, 62.6053) (-52.9378, 63.1629) knots 0 0 0 1 2 2 2
  spline S119 degree 2 poles (-52.9378, 63.1629) (-52.9378, 63.723) (-53.165, 64.2316) (-53.4128, 64.2316) knots 0 0 0 1 2 2 2
  spline S120 degree 2 poles (-53.4128, 64.2316) (-53.6606, 64.2316) (-53.8852, 63.7256) (-53.8852, 63.1629) knots 0 0 0 1 2 2 2
  line L187 (-51.0766, 61.6656) -> (-51.0766, 63.7721)
  line L188 (-51.0766, 63.7721) -> (-51.8123, 63.7721)
  line L189 (-51.8123, 63.7721) -> (-51.8123, 64.2058)
  line L190 (-51.8123, 64.2058) -> (-51.7659, 64.2058)
  spline S121 degree 2 poles (-51.7659, 64.2058) (-51.3632, 64.2058) (-50.994, 64.4562) (-50.963, 64.7479) knots 0 0 0 1 2 2 2
  line L191 (-50.963, 64.7479) -> (-50.47, 64.7479)
  line L192 (-50.47, 64.7479) -> (-50.47, 61.6656)
  line L193 (-50.47, 61.6656) -> (-51.0766, 61.6656)
  line L194 (-49.5278, 62.5433) -> (-49.5278, 63.1345)
  line L195 (-49.5278, 63.1345) -> (-48.3171, 63.1345)
  line L196 (-48.3171, 63.1345) -> (-48.3171, 62.5433)
  line L197 (-48.3171, 62.5433) -> (-49.5278, 62.5433)
  spline S122 degree 2 poles (-48.0486, 63.1629) (-48.0486, 63.9579) (-47.4962, 64.7479) (-46.936, 64.7479) knots 0 0 0 1 2 2 2
  spline S123 degree 2 poles (-46.936, 64.7479) (-46.3784, 64.7479) (-45.8208, 63.9528) (-45.8208, 63.1577) knots 0 0 0 1 2 2 2
  spline S124 degree 2 poles (-45.8208, 63.1577) (-45.8208, 62.3652) (-46.3732, 61.5804) (-46.936, 61.5804) knots 0 0 0 1 2 2 2
  spline S125 degree 2 poles (-46.936, 61.5804) (-47.4962, 61.5804) (-48.0486, 62.3678) (-48.0486, 63.1629) knots 0 0 0 1 2 2 2
  spline S126 degree 2 poles (-47.4084, 63.1629) (-47.4084, 62.6027) (-47.1838, 62.0941) (-46.936, 62.0941) knots 0 0 0 1 2 2 2
  spline S127 degree 2 poles (-46.936, 62.0941) (-46.6882, 62.0941) (-46.461, 62.6053) (-46.461, 63.1629) knots 0 0 0 1 2 2 2
  spline S128 degree 2 poles (-46.461, 63.1629) (-46.461, 63.723) (-46.6882, 64.2316) (-46.936, 64.2316) knots 0 0 0 1 2 2 2
  spline S129 degree 2 poles (-46.936, 64.2316) (-47.1838, 64.2316) (-47.4084, 63.7256) (-47.4084, 63.1629) knots 0 0 0 1 2 2 2
  line L198 (-44.5998, 61.6656) -> (-44.5998, 63.7721)
  line L199 (-44.5998, 63.7721) -> (-45.3355, 63.7721)
  line L200 (-45.3355, 63.7721) -> (-45.3355, 64.2058)
  line L201 (-45.3355, 64.2058) -> (-45.289, 64.2058)
  spline S130 degree 2 poles (-45.289, 64.2058) (-44.8863, 64.2058) (-44.5172, 64.4562) (-44.4862, 64.7479) knots 0 0 0 1 2 2 2
  line L202 (-44.4862, 64.7479) -> (-43.9932, 64.7479)
  line L203 (-43.9932, 64.7479) -> (-43.9932, 61.6656)
  line L204 (-43.9932, 61.6656) -> (-44.5998, 61.6656)
  line L205 (-43.0509, 62.5433) -> (-43.0509, 63.1345)
  line L206 (-43.0509, 63.1345) -> (-41.8402, 63.1345)
  line L207 (-41.8402, 63.1345) -> (-41.8402, 62.5433)
  line L208 (-41.8402, 62.5433) -> (-43.0509, 62.5433)
  line L209 (-40.5805, 64.8356) -> (-39.8267, 64.8356)
  line L210 (-39.8267, 64.8356) -> (-38.6832, 61.6656)
  line L211 (-38.6832, 61.6656) -> (-39.3672, 61.6656)
  line L212 (-39.3672, 61.6656) -> (-39.5841, 62.3187)
  line L213 (-39.5841, 62.3187) -> (-40.8128, 62.3187)
  line L214 (-40.8128, 62.3187) -> (-41.0219, 61.6656)
  line L215 (-41.0219, 61.6656) -> (-41.7086, 61.6656)
  line L216 (-41.7086, 61.6656) -> (-40.5805, 64.8356)
  line L217 (-40.201, 64.2006) -> (-40.6399, 62.8531)
  line L218 (-40.6399, 62.8531) -> (-39.7596, 62.8531)
  line L219 (-39.7596, 62.8531) -> (-40.201, 64.2006)
  point P0 (-5.5793, 57.7464)
  constraints: 2 other
emboss "Emboss1" sketch "Sketch5" operation add depth 0.5 direction (0, 1, 0)
fillet "Fillet4" radius 1 8 edges at (51.4518, 10, 17.9678) (52.0376, 10, -21.9464) (51.4518, 10, -61.8606) (-25.9624, 10, -62.4464) (-103.3766, 10, -61.8606) (-103.9624, 10, -21.9464) (-103.3766, 10, 17.9678) (-25.9624, 10, 18.5536)
equation "\"d1\" = lid_gasket_delta"
equation "\"d2\" = lid_gasket_delta"
equation "\"d3\" = lid_gasket_delta"
equation "\"d8\" = min_wall_width"
equation "\"d6\" = lid_height - wall_thickness"
equation "\"d12\" = pem_height"
equation "\"d14\" = pem_height"
equation "\"d16\" = PEM_fillet"
equation "\"d18\" = lid_screw_d"
equation "\"d23\" = pem_height"
equation "\"d30\" = bottom_fillet"
equation "\"wall_thickness\" = wall_thickness_1"
equation "\"min_wall_width\" = 1"
equation "\"lid_height\" = 10"
equation "\"pem_height\" = 4"
equation "\"PEM_fillet\" = 1.5"
equation "\"lid_screw_d\" = 4"
equation "\"bottom_fillet\" = 1"
equation "\"wall_thickness_1\" = 3"
body "Solid1"
